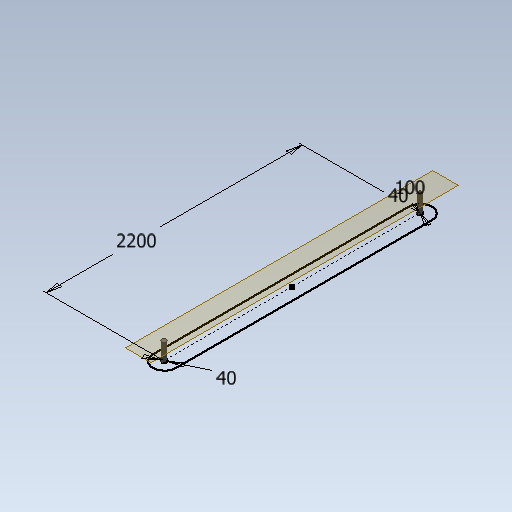
# Autodesk Inventor part: arm j2
Saved by Autodesk Inventor 2020 (Build 240168000, 168)
## iProperties
Created: 2020-07-11
Part Number: arm j2
Material: Aluminum 6061
Document SubType Name: Modeling
Designer: Vikki
Density: 2.7 g/cm^3
Appearance: Glossy - Black
Mass: 1017.88 g
Surface Area: 427.257 cm^2
Volume: 376.991 cm^3
Author: Vikki
Autodesk Inventor part; units mm, degrees
ref_plane "YZ Plane" through (0, 0, 0) normal (1, 0, 0) x (0, 1, 0)
ref_plane "XY Plane" through (0, 0, 0) normal (0, 0, 1) x (1, 0, 0)
sketch "Sketch1" plane through (0, 0, 0) normal (0, 1, 0) x (-1, 0, 0)
  line L0 (0, 0) -> (0, -2200) construction
  line L1 (-100, 0) -> (-100, -2200)
  line L2 (100, -2200) -> (100, 0)
  arc A0 (100, 0) -> (-100, 0) centre (0, 0) ccw
  arc A1 (-100, -2200) -> (100, -2200) centre (0, -2200) ccw
  circle A2 centre (0, 0) radius 20
  circle A3 centre (0, -2200) radius 20
  point P0 (0, -1100)
  dimension "d0" = 2200
  dimension "d1" = 100
  dimension "d2" = 40
  dimension "d3" = 40
  constraints: 8 end point, 4 centre point, 4 point on circle, 4 tangent, 2 coincident, 1 midpoint, 1 parallel, 1 vertical
  measures "d0" distance of L0.start L0.end
  measures "d1" radius of A1
  measures "d2" diameter of A2
  measures "d3" diameter of A3
ref_plane "Work Plane1" through (0, 150, 0) normal (0, 1, 0) x (-1, 0, 0)
sketch "Sketch2" plane through (0, 150, 0) normal (0, 1, 0) x (-1, 0, 0)
  line L0 (100, -2200) -> (100, 0) projected
  arc A0 (-100, -2200) -> (100, -2200) centre (0, -2200) ccw projected
  circle A1 centre (0, -2200) radius 20 projected
  line L1 (-100, 0) -> (-100, -2200) projected
  circle A2 centre (0, 0) radius 20 projected
  arc A3 (100, 0) -> (-100, 0) centre (0, 0) ccw projected
extrude "Extrusion1" add sketch "Sketch2" against normal up to surface (150 mm away) contours A1 | A2
body "Solid1"
